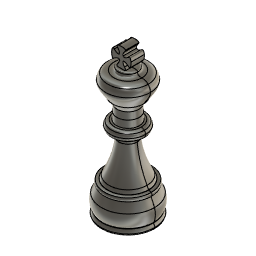
King v1 (Autodesk Fusion 360 design; units mm, degrees)
Autodesk Fusion 360 part; units mm, degrees
sketch "king side view" plane through (0, 0, 0) normal (0, 1, 0) x (1, 0, 0)
  spline S0 degree 3 poles (21.5371, -125.1018) (20.0819, -124.6784) (20.0025, -124.308) (21.0873, -122.9057) knots 0 0 0 0 1 1 1 1
  spline S1 degree 3 poles (21.0873, -122.9057) (21.8281, -121.9532) (22.0663, -121.4241) (22.0663, -120.5509) knots 0 0 0 0 1 1 1 1
  spline S2 degree 3 poles (22.0663, -120.5509) (22.0927, -119.5984) (22.0133, -119.4397) (21.5106, -119.3603) knots 0 0 0 0 1 1 1 1
  spline S3 degree 3 poles (21.5106, -119.3603) (20.7963, -119.2545) (19.1029, -120.1011) (18.2827, -121.0007) knots 0 0 0 0 1 1 1 1
  spline S4 degree 3 poles (18.2827, -121.0007) (17.9123, -121.3711) (17.5419, -121.6886) (17.4625, -121.6886) knots 0 0 0 0 1 1 1 1
  spline S5 degree 3 poles (17.4625, -121.6886) (17.0127, -121.6886) (16.2719, -119.3868) (16.2983, -118.0109) knots 0 0 0 0 1 1 1 1
  spline S6 degree 3 poles (16.2983, -118.0109) (16.2983, -116.4499) (16.801, -114.5449) (17.2244, -114.5449) knots 0 0 0 0 1 1 1 1
  spline S7 degree 3 poles (17.2244, -114.5449) (17.3567, -114.5449) (17.9388, -114.8889) (18.5473, -115.3122) knots 0 0 0 0 1 1 1 1
  spline S8 degree 3 poles (18.5473, -115.3122) (20.6375, -116.8468) (22.225, -116.9261) (22.225, -115.5503) knots 0 0 0 0 1 1 1 1
  spline S9 degree 3 poles (22.225, -115.5503) (22.225, -114.9682) (21.0873, -112.9045) (20.5052, -112.4282) knots 0 0 0 0 1 1 1 1
  spline S10 degree 3 poles (20.5052, -112.4282) (18.9177, -111.1053) (22.7542, -109.9941) (25.8763, -110.8407) knots 0 0 0 0 1 1 1 1
  spline S11 degree 3 poles (25.8763, -110.8407) (26.4848, -110.9995) (26.9875, -111.2376) (26.9875, -111.3964) knots 0 0 0 0 1 1 1 1
  spline S12 degree 3 poles (26.9875, -111.3964) (26.9875, -111.5551) (26.5113, -112.3489) (25.9292, -113.1426) knots 0 0 0 0 1 1 1 1
  spline S13 degree 3 poles (25.9292, -113.1426) (24.8708, -114.6243) (24.5269, -116.1589) (25.1619, -116.5293) knots 0 0 0 0 1 1 1 1
  spline S14 degree 3 poles (25.1619, -116.5293) (25.744, -116.8997) (27.305, -116.3176) (28.4956, -115.2857) knots 0 0 0 0 1 1 1 1
  spline S15 degree 3 poles (28.4956, -115.2857) (29.6598, -114.2803) (29.7656, -114.2539) (30.0831, -114.7036) knots 0 0 0 0 1 1 1 1
  spline S16 degree 3 poles (30.0831, -114.7036) (30.7181, -115.5503) (31.0092, -117.2436) (30.824, -118.7518) knots 0 0 0 0 1 1 1 1
  spline S17 degree 3 poles (30.824, -118.7518) (30.48, -121.4505) (30.0038, -121.7151) (27.94, -120.2334) knots 0 0 0 0 1 1 1 1
  spline S18 degree 3 poles (27.94, -120.2334) (26.4054, -119.1486) (25.5852, -119.0693) (25.0031, -119.9424) knots 0 0 0 0 1 1 1 1
  spline S19 degree 3 poles (25.0031, -119.9424) (24.5269, -120.6832) (24.6063, -120.9214) (25.9556, -122.9322) knots 0 0 0 0 1 1 1 1
  spline S20 degree 3 poles (25.9556, -122.9322) (26.379, -123.5407) (26.7229, -124.2022) (26.7229, -124.4139) knots 0 0 0 0 1 1 1 1
  spline S21 degree 3 poles (26.7229, -124.4139) (26.7229, -125.2605) (23.5215, -125.6839) (21.5371, -125.1018) knots 0 0 0 0 1 1 1 1
  spline S22 degree 3 poles (16.6688, -109.5972) (16.0338, -109.3855) (15.6104, -108.6976) (15.6104, -107.9039) knots 0 0 0 0 1 1 1 1
  spline S23 degree 3 poles (15.6104, -107.9039) (15.6104, -106.8984) (15.2135, -106.6868) (12.9117, -106.528) knots 0 0 0 0 1 1 1 1
  spline S24 degree 3 poles (12.9117, -106.528) (8.3608, -106.2105) (6.1119, -104.1203) (6.0854, -100.2574) knots 0 0 0 0 1 1 1 1
  spline S25 degree 3 poles (6.0854, -100.2574) (6.0854, -97.9291) (6.7204, -96.6591) (11.2448, -89.9651) knots 0 0 0 0 1 1 1 1
  line L0 (11.2448, -89.9651) -> (14.8696, -84.5676)
  line L1 (14.8696, -84.5676) -> (14.6844, -79.9109)
  spline S26 degree 3 poles (14.6844, -79.9109) (14.605, -77.3445) (14.4463, -75.0426) (14.3933, -74.8045) knots 0 0 0 0 1 1 1 1
  spline S27 degree 3 poles (14.3933, -74.8045) (14.2875, -74.4341) (13.97, -74.3282) (13.0704, -74.3282) knots 0 0 0 0 1 1 1 1
  spline S28 degree 3 poles (13.0704, -74.3282) (12.409, -74.3282) (11.5358, -74.143) (11.1125, -73.9314) knots 0 0 0 0 1 1 1 1
  spline S29 degree 3 poles (11.1125, -73.9314) (9.6044, -73.1641) (9.0488, -70.9945) (9.8954, -69.3541) knots 0 0 0 0 1 1 1 1
  spline S30 degree 3 poles (9.8954, -69.3541) (10.7421, -67.7136) (10.7156, -67.7136) (23.2833, -67.7136) knots 0 0 0 0 1 1 1 1
  line L2 (23.2833, -67.7136) -> (34.6604, -67.7136)
  line L3 (34.6604, -67.7136) -> (35.6658, -68.6132)
  spline S31 degree 3 poles (35.6658, -68.6132) (36.5654, -69.4599) (36.6448, -69.6451) (36.6448, -70.9945) knots 0 0 0 0 1 1 1 1
  spline S32 degree 3 poles (36.6448, -70.9945) (36.6448, -72.2909) (36.539, -72.5555) (35.7981, -73.3228) knots 0 0 0 0 1 1 1 1
  spline S33 degree 3 poles (35.7981, -73.3228) (35.1102, -74.0107) (34.6604, -74.1959) (33.5492, -74.3282) knots 0 0 0 0 1 1 1 1
  line L4 (33.5492, -74.3282) -> (32.1469, -74.4605)
  line L5 (32.1469, -74.4605) -> (31.9088, -79.6728)
  line L6 (31.9088, -79.6728) -> (31.6971, -84.8851)
  line L7 (31.6971, -84.8851) -> (35.1102, -89.9916)
  spline S34 degree 3 poles (35.1102, -89.9916) (40.1373, -97.4528) (40.349, -97.8761) (40.349, -100.1251) knots 0 0 0 0 1 1 1 1
  spline S35 degree 3 poles (40.349, -100.1251) (40.3225, -102.1095) (39.9256, -103.2207) (38.6556, -104.5701) knots 0 0 0 0 1 1 1 1
  spline S36 degree 3 poles (38.6556, -104.5701) (37.5708, -105.7607) (36.5654, -106.1576) (33.999, -106.3693) knots 0 0 0 0 1 1 1 1
  spline S37 degree 3 poles (33.999, -106.3693) (31.3796, -106.5809) (30.6917, -107.0307) (30.6917, -108.433) knots 0 0 0 0 1 1 1 1
  spline S38 degree 3 poles (30.6917, -108.433) (30.6917, -109.7559) (30.5329, -109.7824) (23.5744, -109.7559) knots 0 0 0 0 1 1 1 1
  spline S39 degree 3 poles (23.5744, -109.7559) (19.976, -109.7559) (16.8804, -109.6766) (16.6688, -109.5972) knots 0 0 0 0 1 1 1 1
  spline S40 degree 3 poles (16.7746, -66.9993) (16.4835, -66.7876) (16.219, -65.0678) (15.6104, -58.9824) knots 0 0 0 0 1 1 1 1
  spline S41 degree 3 poles (15.6104, -58.9824) (15.2929, -55.7016) (13.8377, -49.0605) (12.8323, -46.2824) knots 0 0 0 0 1 1 1 1
  spline S42 degree 3 poles (12.8323, -46.2824) (12.4354, -45.1976) (11.2183, -42.2872) (10.1335, -39.8266) knots 0 0 0 0 1 1 1 1
  spline S43 degree 3 poles (10.1335, -39.8266) (9.0488, -37.3659) (8.2285, -35.1964) (8.3079, -35.0111) knots 0 0 0 0 1 1 1 1
  spline S44 degree 3 poles (8.3079, -35.0111) (8.4138, -34.6936) (11.0331, -34.6407) (23.6802, -34.6407) knots 0 0 0 0 1 1 1 1
  line L8 (23.6802, -34.6407) -> (38.8937, -34.6407)
  line L9 (38.8938, -34.6407) -> (38.8938, -35.2228)
  spline S45 degree 3 poles (38.8938, -35.2228) (38.8938, -35.5403) (38.444, -36.6251) (37.8619, -37.657) knots 0 0 0 0 1 1 1 1
  spline S46 degree 3 poles (37.8619, -37.657) (33.9725, -44.8272) (31.459, -53.0822) (30.4535, -62.0516) knots 0 0 0 0 1 1 1 1
  spline S47 degree 3 poles (30.4535, -62.0516) (30.189, -64.4593) (29.8185, -66.5759) (29.6598, -66.7347) knots 0 0 0 0 1 1 1 1
  spline S48 degree 3 poles (29.6598, -66.7347) (29.2894, -67.1051) (17.2773, -67.3168) (16.7746, -66.9993) knots 0 0 0 0 1 1 1 1
  spline S49 degree 3 poles (6.4029, -33.6618) (5.4769, -32.868) (5.3975, -31.8626) (6.1913, -31.0953) knots 0 0 0 0 1 1 1 1
  line L10 (6.1913, -31.0953) -> (6.8527, -30.4074)
  line L11 (6.8527, -30.4074) -> (23.6802, -30.4074)
  spline S50 degree 3 poles (23.6802, -30.4074) (40.1373, -30.4074) (40.4813, -30.4074) (41.0104, -30.9366) knots 0 0 0 0 1 1 1 1
  spline S51 degree 3 poles (41.0104, -30.9366) (41.6983, -31.6245) (41.6983, -32.8416) (40.984, -33.4766) knots 0 0 0 0 1 1 1 1
  spline S52 degree 3 poles (40.984, -33.4766) (40.4548, -33.9528) (39.714, -33.9793) (23.6802, -34.0586) knots 0 0 0 0 1 1 1 1
  spline S53 degree 3 poles (23.6802, -34.0586) (7.9904, -34.1116) (6.9056, -34.0851) (6.4029, -33.6618) knots 0 0 0 0 1 1 1 1
  spline S54 degree 3 poles (7.0115, -29.3755) (5.2652, -28.3172) (3.3867, -25.1157) (2.6458, -21.9672) knots 0 0 0 0 1 1 1 1
  spline S55 degree 3 poles (2.6458, -21.9672) (2.1696, -19.9034) (2.4342, -16.6491) (3.2808, -14.4001) knots 0 0 0 0 1 1 1 1
  spline S56 degree 3 poles (3.2808, -14.4001) (4.4715, -11.3045) (2.2225, -11.622) (22.9923, -11.622) knots 0 0 0 0 1 1 1 1
  spline S57 degree 3 poles (22.9923, -11.622) (43.2329, -11.622) (41.8571, -11.4897) (42.8625, -13.4741) knots 0 0 0 0 1 1 1 1
  spline S58 degree 3 poles (42.8625, -13.4741) (44.2648, -16.2257) (44.5029, -20.2209) (43.4181, -23.2636) knots 0 0 0 0 1 1 1 1
  spline S59 degree 3 poles (43.4181, -23.2636) (42.7302, -25.248) (41.0369, -28.8464) (40.5342, -29.4284) knots 0 0 0 0 1 1 1 1
  spline S60 degree 3 poles (40.5342, -29.4284) (40.1638, -29.8518) (39.026, -29.8782) (23.9713, -29.8782) knots 0 0 0 0 1 1 1 1
  spline S61 degree 3 poles (23.9713, -29.8782) (8.7048, -29.8782) (7.7523, -29.8518) (7.0115, -29.3755) knots 0 0 0 0 1 1 1 1
  spline S62 degree 3 poles (4.2069, -10.6959) (3.3338, -10.2197) (2.8575, -9.082) (2.9633, -7.7591) knots 0 0 0 0 1 1 1 1
  line L12 (2.9633, -7.7591) -> (3.0427, -6.7272)
  line L13 (3.0427, -6.7272) -> (22.9923, -6.6478)
  spline S63 degree 3 poles (22.9923, -6.6478) (37.5179, -6.6214) (43.0477, -6.6743) (43.2858, -6.8859) knots 0 0 0 0 1 1 1 1
  spline S64 degree 3 poles (43.2858, -6.8859) (43.4975, -7.0447) (43.6563, -7.468) (43.6563, -7.8384) knots 0 0 0 0 1 1 1 1
  spline S65 degree 3 poles (43.6563, -7.8384) (43.6563, -8.6851) (42.7038, -10.4843) (42.0952, -10.8282) knots 0 0 0 0 1 1 1 1
  spline S66 degree 3 poles (42.0952, -10.8282) (41.7513, -11.0134) (35.3748, -11.0928) (23.2304, -11.0928) knots 0 0 0 0 1 1 1 1
  spline S67 degree 3 poles (23.2304, -11.0928) (7.911, -11.0664) (4.789, -11.0134) (4.2069, -10.6959) knots 0 0 0 0 1 1 1 1
  line L14 (23.5744, -109.7559) -> (23.5744, -6.6468)
  constraint coincident S63 L14.end
  constraint vertical L14
revolve "Revolve1" add sketch "king side view" angle 360 about axis through (23.5744, 0, 109.7559) along (0, 0, -1) contours L2 L3 S31 S32 S33 L4 L5 L6 L7 S34 S35 S36 S37 S38 L14 | S44 L8 L9 S45 S46 S47 S48 L14 | L11 S50 S51 S52 S53 L14 | S57 S58 S59 S60 S61 L14 | S63 S64 S65 S66 L14 makes body 1 at (35.0536, 6.2512, 30.44) makes body 2 at (15.6506, -7.9362, 44.2593) makes body 3 at (4.0498, -6.0225, 20.6679) makes body 4 at (10.6498, 8.8118, 96.2902) makes body 5 at (13.882, -8.7709, 6.6612)
extrude "Extrude1" add sketch "king side view" along normal blind 5 and the other way blind 5 separate body contours S0 S1 S2 S3 S4 S5 S6 S7 S8 S9 S10 S11 S12 S13 S14 S15 S16 S17 S18 S19 S20 S21 makes body 6
move_body "Align1" bodies 3 to x (1, 0, 0) y (0, 1, 0) z (0, 0, 1) at (0, 0, -2.6458)
move_body "Align2" bodies 1 to x (1, 0, 0) y (0, 1, 0) z (0, 0, 1) at (0, 0, -4.154)
move_body "Align3" bodies 2 to x (1, 0, 0) y (0, 1, 0) z (0, 0, 1) at (0, 0, -5.3181)
move_body "Align4" bodies 4 to x (1, 0, 0) y (0, 1, 0) z (0, 0, 1) at (0, 0, -6.2971)
move_body "Move1" bodies 6 to x (1, 0, 0) y (0, 1, 0) z (0, 0, 1) at (0, 0, -7.5)
combine "Combine1" operation add target body 1 tool bodies 2 3 4 5 6
named bodies: "king"
